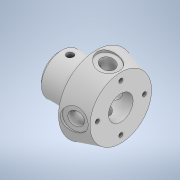
# Autodesk Inventor part: Гайка-7
Saved by Autodesk Inventor 2022 (Build 260153000, 153)
## iProperties
Created: 2021-12-02
Part Number: Гайка-7
Material: Типовые
Document SubType Name: Modeling
Designer: Украинцев
Density: 1 g/cm^3
Appearance: По умолчанию
Author: Украинцев
Autodesk Inventor part; units mm, degrees
ref_plane "YZ Plane" through (0, 0, 0) normal (1, 0, 0) x (0, 1, 0)
ref_plane "XZ Plane" through (0, 0, 0) normal (0, 1, 0) x (-1, 0, 0)
ref_plane "XY Plane" through (0, 0, 0) normal (0, 0, 1) x (1, 0, 0)
sketch "Эскиз1" plane through (0, 0, 0) normal (0, 1, 0) x (-1, 0, 0)
  line L0 (0, 0) -> (0, -22.5)
  line L1 (0, -22.5) -> (18, -22.5)
  line L2 (18, 0) -> (18, -27.5)
  line L3 (18, -27.5) -> (0, -22.5)
  line L4 (0, 0) -> (45, 0)
  line L5 (45, 0) -> (45, -15)
  line L6 (45, -15) -> (25, -15)
  line L7 (25, -15) -> (18, -27.5)
  line L8 (9, -25) -> (18.679145, 11.123061)
  line L9 (9, -25) -> (46.397344, -25) construction
  line L10 (9, -25) -> (9.517638, -23.068148)
  line L11 (9.517638, -23.068148) -> (17.486526, -25.203405)
  line L12 (1.63798, -22.954995) -> (2.155619, -21.023143)
  line L13 (1.63798, -22.954995) -> (3.63798, -22.954995) construction
  line L14 (2.155619, -21.023143) -> (9.517638, -23.068148)
  line L15 (17.486526, -25.203405) -> (16.949355, -27.208154)
  line L16 (9.517638, -23.068148) -> (4.700049, -21.729929)
  line L17 (4.700049, -21.729929) -> (13.502082, 9.957392)
  line L18 (13.502082, 9.957392) -> (23.137261, 7.280953)
  line L19 (23.137261, 7.280953) -> (14.347469, -24.362298)
  point P0 (1.759896, -22.5)
  point P1 (21.114774, 0)
  point P2 (15.69873, 0)
  dimension "d0" = 22.5
  dimension "d3" = 45
  dimension "d4" = 15
  dimension "d5" = 20
  dimension "d6" = 75
  dimension "d7" = 2
  dimension "d8" = 8.25
  dimension "d9" = 2
  dimension "d10" = 75
  dimension "d11" = 5
  dimension "d12" = 10
  constraints: 40 end point, 6 perpendicular, 4 point on line, 3 horizontal, 2 equal length, 2 vertical, 1 midpoint
  measures "d0" distance of L0.start L0.end
  measures "d3" distance of L0.start L4.end
  measures "d4" distance of L4.end L5.end
  measures "d5" distance of L5.end L6.end
  measures "d6" angle of L9 L8
  measures "d7" distance of L8.start L10.end
  measures "d8" distance of L10.end L11.end
  measures "d9" distance of L12.start L12.end
  measures "d10" angle of L13 L12
  measures "d11" distance of L10.end L16.end
  measures "d12" distance of L17.end L18.end
sketch "Эскиз1 outline for Вращение1" plane through (0, 0, 0) normal (0, 1, 0) x (-1, 0, 0)
  line L0 (18, -27.5) -> (25, -15)
  line L1 (25, -15) -> (45, -15)
  line L2 (45, -15) -> (45, 0)
  line L3 (45, 0) -> (0, 0)
  line L4 (0, 0) -> (0, -22.5)
  line L5 (0, -22.5) -> (18, -27.5)
revolve "Вращение1" add sketch "Эскиз1 outline for Вращение1" angle 360 about axis through (0, 0, 0) along (-1, 0, 0)
sketch "Эскиз2" plane through (0, 0, 0) normal (1, 0, 0) x (0, 0, -1)
  point P0 (0, 0)
  point P1 (0, 0)
  constraints: 1 coincident
hole "Отверстие1" at (0, 0, 0) direction (-1, 0, 0) diameter 14.8 end through all counterbore diameter 18 counterbore depth 23
sketch "Эскиз1 outline for Вращение2" plane through (0, 0, 0) normal (0, 1, 0) x (-1, 0, 0)
  line L0 (16.949355, -27.208154) -> (17.486526, -25.203405)
  line L1 (9, -25) -> (16.949355, -27.208154)
  line L2 (15.69873, 0) -> (9, -25)
  line L3 (21.114774, 0) -> (15.69873, 0)
  line L4 (14.347469, -24.362298) -> (21.114774, 0)
  line L5 (17.486526, -25.203405) -> (14.347469, -24.362298)
revolve "Вращение2" cut sketch "Эскиз1 outline for Вращение2" angle 360 about axis through (-9, 0, -25) along (-0.258819, 0, 0.9659258)
pattern_circular "Круговой массив1" count 4 over 360 about axis through (-21.5, 0, 0) along (1, 0, 0) of "Вращение2"
sketch "Эскиз3" plane through (0, 0, 0) normal (1, 0, 0) x (0, 0, -1)
  line L0 (0, 0) -> (0, -17.2)
  circle A0 centre (0, -17.2) radius 1.5
  dimension "d25" = 17.2
  dimension "d26" = 3
  constraints: 2 end point, 1 centre point, 1 coincident, 1 vertical
  measures "d25" distance of L0.start L0.end
  measures "d26" diameter of A0
sketch "Эскиз3 outline for Выдавливание1" plane through (0, 0, 0) normal (1, 0, 0) x (0, 0, -1)
  circle A0 centre (0, -17.2) radius 1.5
extrude "Выдавливание1" cut sketch "Эскиз3 outline for Выдавливание1" against normal through all
pattern_circular "Круговой массив2" count 4 over 360 about axis through (-9, 0, 0) along (1, 0, 0) of "Выдавливание1"
sketch "Эскиз4" plane through (0, 0, 0) normal (0, 1, 0) x (-1, 0, 0)
  line L0 (45, 15) -> (45, -15) projected
  line L1 (45, 0) -> (37, 0)
  circle A0 centre (37, 0) radius 2.5
  point P0 (0, 0)
  dimension "d32" = 8
  dimension "d33" = 5
  constraints: 2 end point, 1 centre point, 1 coincident, 1 horizontal, 1 midpoint
  measures "d32" distance of L1.start L1.end
  measures "d33" diameter of A0
sketch "Эскиз4 outline for Выдавливание2" plane through (0, 0, 0) normal (0, 1, 0) x (-1, 0, 0)
  circle A0 centre (37, 0) radius 2.5
extrude "Выдавливание2" cut sketch "Эскиз4 outline for Выдавливание2" along normal through all both and the other way through all
chamfer "Фаска1" distance 1.6 angle 45 2 edges at (-23, 0, 7.4) (-45, 0, 7.4)
chamfer "Фаска2" distance 2 angle 45 1 edges at (-45, 0, 15)
